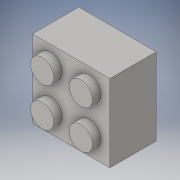
# Autodesk Inventor part: Yee_2x2Brick
Saved by Autodesk Inventor 2016 (Build 200138000, 138)
## iProperties
Created: 2018-02-11
Part Number: Yee_2x2Brick
Material: Generic
Document SubType Name: Modeling
Designer: Nathan
Density: 1 g/cm^3
Appearance: Default
Author: Nathan
Autodesk Inventor part; units mm, degrees
ref_plane "YZ Plane" through (0, 0, 0) normal (1, 0, 0) x (0, 1, 0)
ref_plane "XZ Plane" through (0, 0, 0) normal (0, 1, 0) x (-1, 0, 0)
ref_plane "XY Plane" through (0, 0, 0) normal (0, 0, 1) x (1, 0, 0)
sketch "Sketch1" plane through (0, 0, 0) normal (0, 0, 1) x (1, 0, 0)
  line L0 (0, 0) -> (16, 0)
  line L1 (16, 0) -> (16, 16)
  line L2 (16, 16) -> (0, 16)
  line L3 (0, 16) -> (0, 0)
  dimension "d0" = 16
  dimension "d1" = 16
  constraints: 8 end point, 2 parallel, 1 horizontal, 1 perpendicular
  measures "d0" distance of L2.end L1.end
  measures "d1" distance of L1.end L0.end
extrude "Extrusion1" add sketch "Sketch1" against normal blind 9.6
sketch "Sketch2" plane through (0, 0, 0) normal (0, 0, 1) x (1, 0, 0)
  circle A0 centre (3.8, 12.2) radius 2.4
  line L0 (0, 16) -> (0, 0) projected
  line L1 (16, 16) -> (0, 16) projected
  circle A1 centre (11.8, 12.2) radius 2.4
  circle A2 centre (3.8, 4.2) radius 2.4
  circle A3 centre (11.8, 4.2) radius 2.4
  dimension "d4" = 4.8
  dimension "d5" = 3.8
  dimension "d6" = 3.8
  dimension "d7" = 4.8
  dimension "d8" = 8
  dimension "d9" = 4.8
  dimension "d10" = 4.8
  dimension "d11" = 8
  constraints: 4 centre point, 2 horizontal alignment, 2 vertical alignment
  measures "d4" diameter of A0
  measures "d5" distance from line of L0 A0.centre
  measures "d6" distance from line of L1 A0.centre
  measures "d7" diameter of A1
  measures "d8" distance of A1.centre A0.centre
  measures "d9" diameter of A2
  measures "d10" diameter of A3
  measures "d11" distance of A2.centre A0.centre
extrude "Extrusion2" add sketch "Sketch2" along normal blind 1.8
sketch "Sketch3" plane through (0, 0, -9.6) normal (0, 0, -1) x (-1, 0, 0)
  line L0 (-14.8, 14.8) -> (-1.2, 14.8)
  line L1 (-1.2, 14.8) -> (-1.2, 1.2)
  line L2 (-1.2, 1.2) -> (-14.8, 1.2)
  line L3 (-14.8, 1.2) -> (-14.8, 14.8)
  line L4 (0, 16) -> (-16, 16) projected
  line L5 (-16, 16) -> (-16, 0) projected
  line L6 (-16, 0) -> (0, 0) projected
  line L7 (0, 16) -> (0, 0) projected
  circle A0 centre (-8, 8) radius 3.25
  circle A1 centre (-8, 8) radius 2.4
  dimension "d14" = 1.2
  dimension "d15" = 1.2
  dimension "d16" = 1.2
  dimension "d17" = 1.2
  dimension "d18" = 6.5
  dimension "d19" = 8
  dimension "d20" = 8
  dimension "d21" = 4.8
  constraints: 8 end point, 2 centre point, 2 parallel, 1 coincident, 1 horizontal, 1 perpendicular
  measures "d14" distance between parallel lines of L4 L0
  measures "d15" distance between parallel lines of L5 L3
  measures "d16" distance between parallel lines of L6 L2
  measures "d17" distance between parallel lines of L7 L1
  measures "d18" diameter of A0
  measures "d19" distance from line of L5 A0.centre
  measures "d20" distance from line of L4 A0.centre
  measures "d21" diameter of A1
extrude "Extrusion3" cut sketch "Sketch3" against normal blind 8.4 contours L0 L1 L2 L3 | A1
body "Solid1"
